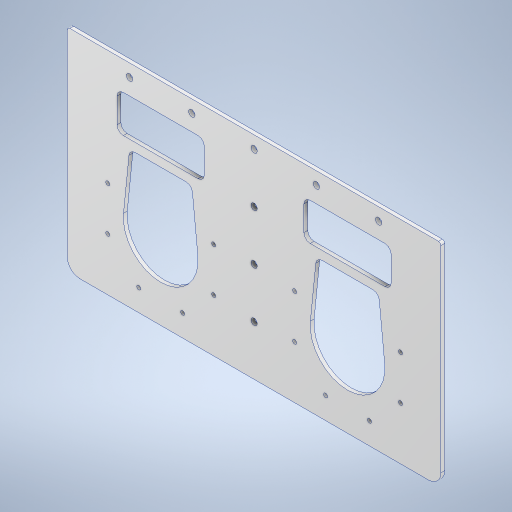
# Autodesk Inventor part: RP_Waist-Under-ver2
Saved by Autodesk Inventor 2024.3 (Build 283343000, 343)
## iProperties
Created: 2025-05-05
Part Number: RP_Waist-Under-ver2
Material: アルミニウム 6061
Document SubType Name: Modeling
Designer: 佐藤智貴
Density: 2.7 g/cm^3
Appearance: アルミニウム - フラット
Mass: 322.185 g
Surface Area: 851.796 cm^2
Volume: 119.328 cm^3
Author: 佐藤智貴
Autodesk Inventor part; units mm, degrees
ref_plane "YZ Plane" through (0, 0, 0) normal (1, 0, 0) x (0, 1, 0)
ref_plane "XZ Plane" through (0, 0, 0) normal (0, 1, 0) x (-1, 0, 0)
ref_plane "XY Plane" through (0, 0, 0) normal (0, 0, 1) x (1, 0, 0)
sketch "スケッチ1" plane through (0, 0, 0) normal (0, 0, 1) x (1, 0, 0)
  line L0 (0, 0) -> (300, 0)
  line L1 (300, 0) -> (300, 175)
  line L2 (300, 175) -> (0, 175)
  line L3 (0, 175) -> (0, 0)
  dimension "d0" = 175
  dimension "d1" = 300
  constraints: 8 end point, 2 parallel, 1 horizontal, 1 perpendicular
  measures "d0" distance between parallel lines of L0 L2
  measures "d1" distance of L1.end L2.end
extrude "押し出し1" add sketch "スケッチ1" along normal blind 3
sketch "スケッチ2" plane through (0, 0, 3) normal (0, 0, 1) x (1, 0, 0)
  line L0 (-6.3861, 0) -> (323.6139, 0)
  circle A0 centre (75, 60) radius 46
  circle A1 centre (225, 60) radius 46
  line L1 (75, 60) -> (75, 156.1238)
  line L2 (225, 60) -> (225, 147.3766)
  line L3 (75, 60) -> (50.2691, 119.7057)
  line L4 (225, 60) -> (203.3576, 112.2494)
  circle A2 centre (57.3966, 102.4985) radius 1.6
  circle A3 centre (207.3966, 102.4985) radius 1.6
  circle A4 centre (32.5015, 77.6034) radius 1.6
  circle A5 centre (32.5015, 42.3966) radius 1.6
  circle A6 centre (57.3966, 17.5015) radius 1.6
  circle A7 centre (92.6034, 17.5015) radius 1.6
  circle A8 centre (117.4985, 42.3966) radius 1.6
  circle A9 centre (117.4985, 77.6034) radius 1.6
  circle A10 centre (92.6034, 102.4985) radius 1.6
  circle A11 centre (182.5015, 77.6034) radius 1.6
  circle A12 centre (182.5015, 42.3966) radius 1.6
  circle A13 centre (207.3966, 17.5015) radius 1.6
  circle A14 centre (242.6034, 17.5015) radius 1.6
  circle A15 centre (267.4985, 42.3966) radius 1.6
  circle A16 centre (267.4985, 77.6034) radius 1.6
  circle A17 centre (242.6034, 102.4985) radius 1.6
  circle A18 centre (75, 60) radius 30
  circle A19 centre (225, 60) radius 30
  line L5 (323.6139, 175) -> (-6.3861, 175)
  line L6 (-6.3861, 145) -> (19.1813, 0)
  line L7 (323.6139, 145) -> (298.0465, 0)
  line L8 (0, 175) -> (0, 0)
  line L9 (300, 175) -> (300, 0)
  line L10 (300, 175) -> (0, 175) projected
  line L11 (0, 175) -> (0, 0) projected
  dimension "d10" = 92
  dimension "d11" = 92
  dimension "d8" = 60
  dimension "d9" = 60
  dimension "d12" = 22.5
  dimension "d13" = 22.5
  dimension "d14" = 3.2
  dimension "d15" = 3.2
  dimension "d16" = 360
  dimension "d17" = 360
  dimension "d18" = 60
  dimension "d19" = 60
  dimension "d20" = 175
  dimension "d21" = 30
  dimension "d22" = 30
  dimension "d23" = 80
  dimension "d24" = 80
  dimension "d25" = 300
  dimension "d26" = 0
  dimension "d27" = 0
  dimension "d28" = 150
  dimension "d29" = 75
  constraints: 20 end point, 18 centre point, 8 point on line, 2 perpendicular, 2 vertical, 1 coincident, 1 horizontal, 40 other
  measures "d8" distance from line of L0 L1.start
  measures "d9" distance from line of L0 L2.start
  measures "d12" angle of L1 L3
  measures "d13" angle of L2 L4
  measures "d14" diameter of A2
  measures "d15" diameter of A3
  measures "d18" diameter of A18
  measures "d19" diameter of A19
  measures "d20" distance between parallel lines of L0 L5
  measures "d21" distance from line of L5 L6.start
  measures "d22" distance from line of L5 L7.start
  measures "d23" angle of L0 L6
  measures "d24" angle of L0 L7
  measures "d25" distance between parallel lines of L9 L8
  measures "d26" distance between parallel lines of L10 L5
  measures "d27" distance between parallel lines of L11 L8
  measures "d28" distance of L2.start A18.centre
  measures "d29" distance from line of L9 L2.start
extrude "押し出し2" cut sketch "スケッチ2" against normal blind 5 contours A9 A0 | A0 A9 | A8 A0 | A0 A8 | A7 A0 | A0 A7 | A6 A0 | A0 A6 | A18 L3 L1 | L1 L3 A18 | A5 A0 | A0 A5 | A4 A0 | A0 A4 | A16 A1 | A1 A16 | A15 A1 | A1 A15 | A14 A1 | A1 A14 | A13 A1 | A1 A13 | A19 L4 L2 | L2 L4 A19 | A12 A1 | A1 A12 | A11 A1 | A1 A11
sketch "スケッチ3" plane through (0, 0, 3) normal (0, 0, 1) x (1, 0, 0)
  circle A0 centre (75, 60) radius 30 projected
  line L0 (75, 60) -> (100, 60)
  line L1 (100, 60) -> (100, 110)
  line L2 (100, 110) -> (75, 110)
  line L3 (75, 110) -> (75, 60)
  line L4 (75, 110) -> (50, 110)
  line L5 (50, 110) -> (50, 60)
  line L6 (50, 60) -> (75, 60)
  line L7 (75, 60) -> (75, 110)
  line L8 (50, 110) -> (42.3811, 36.1629)
  line L9 (100, 110) -> (107.6189, 36.1629)
  line L10 (300, 175) -> (0, 175) projected
  line L11 (150, 175) -> (150, 0)
  line L12 (0, 0) -> (300, 0) projected
  line L13 (200, 110) -> (225, 110)
  line L14 (225, 110) -> (250, 110)
  line L15 (250, 110) -> (257.6189, 36.1629)
  line L16 (200, 110) -> (192.3811, 36.1629)
  circle A1 centre (225, 60) radius 30 projected
  circle A2 centre (225, 60) radius 30
  point P0 (45.1584, 63.0792)
  point P1 (104.8416, 63.0792)
  point P2 (195.1584, 63.0792)
  point P3 (254.8416, 63.0792)
  dimension "d32" = 25
  dimension "d33" = 50
  dimension "d34" = 25
  constraints: 30 end point, 6 symmetric about line, 4 parallel, 2 horizontal, 2 midpoint, 2 perpendicular, 1 centre point, 1 coincident, 1 tangent
  measures "d32" distance of L1.end L2.end
  measures "d33" distance of L0.end L1.end
  measures "d34" distance between parallel lines of L5 L3
extrude "押し出し3" cut sketch "スケッチ3" against normal blind 5 contours A0 L1 L9 | L8 L5 A0 | A0 L3 L2 L1 | L5 L4 L3 A0 | L13 L14 L15 A1 L16
sketch "スケッチ4" plane through (0, 0, 3) normal (0, 0, 1) x (1, 0, 0)
  line L0 (0, 175) -> (0, 0) projected
  line L1 (300, 0) -> (300, 175) projected
  line L2 (0, 175) -> (300, 175)
  line L3 (300, 175) -> (300, 110)
  line L4 (300, 110) -> (0, 110)
  line L5 (0, 110) -> (0, 175)
  line L6 (0, 147) -> (300, 147)
  line L7 (300, 147) -> (300, 117)
  line L8 (300, 117) -> (0, 117)
  line L9 (0, 117) -> (0, 147)
  line L10 (40, 147) -> (110, 147)
  line L11 (110, 147) -> (110, 117)
  line L12 (110, 117) -> (40, 117)
  line L13 (40, 117) -> (40, 147)
  line L14 (150, 117) -> (150, 0)
  line L15 (190, 147) -> (190, 117)
  line L16 (260, 117) -> (260, 147)
  point P0 (110, 147)
  dimension "d38" = 65
  dimension "d39" = 30
  dimension "d40" = 7
  dimension "d41" = 70
  dimension "d192" = 40
  constraints: 30 end point, 6 parallel, 5 point on line, 4 symmetric about line, 3 horizontal, 3 perpendicular, 1 midpoint, 1 vertical
  measures "d38" distance between parallel lines of L2 L4
  measures "d39" distance from line of L14.start L6
  measures "d40" distance between parallel lines of L4 L8
  measures "d41" distance between parallel lines of L11 L13
  measures "d192" distance between parallel lines of L14 L11
extrude "押し出し4" cut sketch "スケッチ4" against normal blind 5 contours L6 L11 L8 L13 | L16 L8 L15 L6
fillet "フィレット2" radius 5 12 edges at (110, 147, 1.5) (260, 147, 1.5) (260, 117, 1.5) (190, 147, 1.5) (190, 117, 1.5) (40, 117, 1.5) (40, 147, 1.5) (110, 117, 1.5) (100, 110, 1.5) (250, 110, 1.5) (200, 110, 1.5) (50, 110, 1.5)
sketch "スケッチ5" plane through (0, 0, 3) normal (0, 0, 1) x (1, 0, 0)
  line L0 (300, 175) -> (0, 175) projected
  line L1 (300, 0) -> (300, 175) projected
  line L2 (0, 175) -> (300, 175)
  line L3 (300, 175) -> (300, 170)
  line L4 (300, 170) -> (0, 170)
  line L5 (0, 170) -> (0, 175)
  line L6 (20, 175) -> (20, 170)
  line L7 (40, 175) -> (40, 170)
  line L8 (60, 175) -> (60, 170)
  line L9 (80, 175) -> (80, 170)
  line L10 (100, 175) -> (100, 170)
  line L11 (120, 175) -> (120, 170)
  line L12 (140, 175) -> (140, 170)
  line L13 (160, 175) -> (160, 170)
  line L14 (180, 175) -> (180, 170)
  line L15 (200, 175) -> (200, 170)
  line L16 (220, 175) -> (220, 170)
  line L17 (240, 175) -> (240, 170)
  line L18 (260, 175) -> (260, 170)
  line L19 (280, 175) -> (280, 170)
  line L20 (300, 175) -> (300, 170)
  point P0 (0, 0)
  point P1 (0, 172.5)
  dimension "d46" = 5
  dimension "d47" = 20
  dimension "d50" = 20
  constraints: 38 end point, 3 point on line, 2 horizontal, 2 parallel, 2 perpendicular, 1 midpoint, 42 other
  measures "d46" distance between parallel lines of L0 L4
  measures "d47" distance from line of point (0, 172.5) L6
  measures "d50" distance of L6.start L7.start
extrude "押し出し5" cut sketch "スケッチ5" against normal blind 5
fillet "フィレット6" radius 10 2 edges at (0, 0, 1.5) (300, 0, 1.5)
fillet "フィレット7" radius 2 2 edges at (300, 170, 1.5) (0, 170, 1.5)
sketch "スケッチ12" plane through (0, 0, 3) normal (0, 0, 1) x (1, 0, 0)
  line L0 (298, 170) -> (2, 170) projected
  line L1 (150, 170) -> (150, 0)
  line L2 (10, 0) -> (290, 0) projected
  line L3 (300, 10) -> (300, 168) projected
  line L4 (0, 168) -> (0, 10) projected
  point P0 (0, 0)
  point P1 (150, 40)
  point P2 (150, 80)
  point P3 (150, 120)
  dimension "d194" = 300
  dimension "d195" = 150
  dimension "d196" = 40
  dimension "d197" = 40
  dimension "d198" = 40
  constraints: 3 point on line, 2 end point, 2 midpoint
  measures "d194" distance between parallel lines of L3 L4
  measures "d195" distance between parallel lines of L4 L1
  measures "d196" distance from line of L2 point (150, 40)
  measures "d197" distance of point (150, 40) point (150, 80)
  measures "d198" distance of point (150, 80) point (150, 120)
hole "穴3" at (150, 40, 3) at (150, 80, 3) at (150, 120, 3) direction (0, 0, -1) diameter 5.2 end through all
sketch "スケッチ14" plane through (0, 0, 0) normal (0, 0, -1) x (-1, 0, 0)
  line L0 (-300, 10) -> (-300, 168) projected
  line L1 (-300, 160) -> (0, 160)
  line L2 (0, 168) -> (0, 10) projected
  line L3 (-2, 170) -> (-298, 170) projected
  point P0 (0, 0)
  point P1 (-150, 160)
  point P2 (-200, 160)
  point P3 (-250, 160)
  point P4 (-100, 160)
  point P5 (-50, 160)
  dimension "d220" = 10
  dimension "d221" = 150
  dimension "d222" = 50
  dimension "d223" = 50
  dimension "d224" = 50
  dimension "d225" = 50
  constraints: 6 point on line, 2 end point, 1 horizontal, 1 midpoint
  measures "d220" distance between parallel lines of L3 L1
  measures "d221" distance from line of L0 point (-150, 160)
  measures "d222" distance of point (-200, 160) point (-150, 160)
  measures "d223" distance of point (-200, 160) point (-250, 160)
  measures "d224" distance of point (-150, 160) point (-100, 160)
  measures "d225" distance of point (-100, 160) point (-50, 160)
hole "穴4" at (150, 160, 0) at (200, 160, 0) at (250, 160, 0) at (100, 160, 0) at (50, 160, 0) direction (0, 0, 1) diameter 5.2 end through all
equation "\"d11\" = d10"
equation "\"d8\" = d9"
equation "\"d15\" = d14"
equation "\"d24\" = d23"
equation "\"d34\" = d32"
